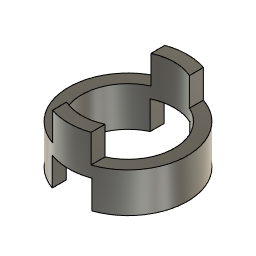
spacer v2 (Autodesk Fusion 360 design; units mm, degrees)
Autodesk Fusion 360 part; units mm, degrees
note: some values were not read from the file. Set by a fixed rule: which sketch regions a step uses.
sketch "Sketch1" plane through (0, 0, 0) normal (0, 0, 1) x (1, 0, 0)
  circle A0 centre (0, 0) radius 5.25
  circle A1 centre (0, 0) radius 4.1
  dimension "d1" = 10.5
  dimension "d2" = 8.2
  constraint coincident A0.centre A1.centre
  constraint concentric A0 A1
  measures "d1" diameter of A0
  measures "d2" diameter of A1
extrude "Extrude1" add sketch "Sketch1" along normal blind 6
sketch "Sketch2" plane through (0, 0, 0) normal (0, 0, -1) x (1, 0, 0)
  circle A0 centre (0, 0) radius 4.1
  circle A1 centre (0, 0) radius 5.25
  line L0 (-1.75, 6.7486) -> (1.75, 6.7486)
  line L1 (1.75, 6.7486) -> (1.75, -6.7486)
  line L2 (1.75, -6.7486) -> (-1.75, -6.7486)
  line L3 (-1.75, -6.7486) -> (-1.75, 6.7486)
  line L4 (-1.75, 6.7486) -> (1.75, -6.7486) construction
  line L5 (1.75, 6.7486) -> (-1.75, -6.7486) construction
  dimension "d5" = 3.5
  constraint horizontal L0
  constraint perpendicular L0 L1
  constraint parallel L0 L2
  constraint parallel L1 L3
  constraint coincident L4 A0.centre
  constraint coincident L5 A0.centre
  constraint coincident A0.centre A1.centre
  measures "d5" distance of L1.end L2.end
extrude "Extrude2" cut sketch "Sketch2" against normal blind 2.5 contours A0 A1 L1 L3 | A0 A1 L1 L3
sketch "Sketch3" plane through (0, 0, 6) normal (0, 0, 1) x (-1, 0, 0)
  circle A0 centre (0, 0) radius 4.1
  circle A1 centre (0, 0) radius 5.25
  line L0 (-1.7, -5.9064) -> (1.7, -5.9064)
  line L1 (1.7, -5.9064) -> (1.7, 5.9064)
  line L2 (1.7, 5.9064) -> (-1.7, 5.9064)
  line L3 (-1.7, 5.9064) -> (-1.7, -5.9064)
  line L4 (-1.7, -5.9064) -> (1.7, 5.9064) construction
  line L5 (1.7, -5.9064) -> (-1.7, 5.9064) construction
  dimension "d8" = 3.4
  constraint horizontal L0
  constraint perpendicular L0 L1
  constraint parallel L0 L2
  constraint parallel L1 L3
  constraint coincident L4 A0.centre
  constraint coincident L5 A0.centre
  constraint coincident A0.centre A1.centre
  measures "d8" distance of L1.end L2.end
extrude "Extrude3" cut sketch "Sketch3" against normal blind 2.5 contours A0 A1 L1 | A0 A1 L3
